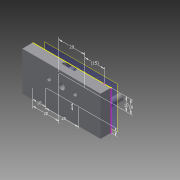
# Autodesk Inventor part: detalKKoretke
Saved by Autodesk Inventor 2015 (Build 190159000, 159)
## iProperties
Created: 2016-04-08
Part Number: detalKKoretke
Material: Generic
Document SubType Name: Modeling
Designer: Andreas
Density: 1 g/cm^3
Appearance: Default
Author: Andreas
Autodesk Inventor part; units mm, degrees
ref_plane "YZ Plane" through (0, 0, 0) normal (1, 0, 0) x (0, 1, 0)
ref_plane "XZ Plane" through (0, 0, 0) normal (0, 1, 0) x (-1, 0, 0)
ref_plane "XY Plane" through (0, 0, 0) normal (0, 0, 1) x (1, 0, 0)
sketch "Sketch1" plane through (0, 0, 0) normal (0, 1, 0) x (-1, 0, 0)
  line L0 (0, 0) -> (60, 0)
  line L1 (60, 0) -> (60, -30)
  line L2 (60, -30) -> (0, -30)
  line L3 (0, -30) -> (0, 0)
  dimension "d0" = 60
  dimension "d1" = 30
  dimension "d2" = 60
  constraints: 8 end point, 2 perpendicular, 1 horizontal
  measures "d0" distance of L0.start L0.end
  measures "d1" distance of L0.end L1.end
  measures "d2" distance of L1.end L2.end
extrude "Extrusion1" add sketch "Sketch1" against normal blind 5 and the other way blind 3
sketch "Sketch2" plane through (0, 3, 0) normal (0, 1, 0) x (1, 0, 0)
  line L0 (-60, 30) -> (-60, 0) projected
  line L1 (0, 0) -> (0, 30) projected
  line L2 (0, 30) -> (-60, 30) projected
  line L3 (-60, 0) -> (0, 0) projected
  line L4 (-5, 0) -> (-5, 30) projected
  point P0 (-40, 10)
  point P1 (-20, 10)
  dimension "d44" = 10
  dimension "d45" = 20
  dimension "d46" = 20
  dimension "d47" = 10
  dimension "d67" = 15
  measures "d44" distance from line of L3 point (-40, 10)
  measures "d45" distance from line of L0 point (-40, 10)
  measures "d46" distance of point (-40, 10) point (-20, 10)
  measures "d47" distance from line of L3 point (-20, 10)
  measures "d67" distance from line of L4 point (-20, 10)
sketch "Sketch3" plane through (0, 3, 0) normal (0, 1, 0) x (1, 0, 0)
  line L0 (0, 30) -> (-60, 30) projected
  line L1 (-60, 0) -> (-60, 30) projected
  point P0 (0, 0)
  point P1 (-50, 25)
  point P2 (-5, 30)
  point P3 (-25, 25)
  dimension "d56" = 5
  dimension "d57" = 10
  dimension "d58" = 25
  dimension "d59" = 5
  measures "d56" distance from line of L0 point (-50, 25)
  measures "d57" distance from line of L1 point (-50, 25)
  measures "d58" distance of point (-50, 25) point (-25, 25)
  measures "d59" distance from line of L0 point (-25, 25)
sketch "Sketch11" plane through (0, 3, 0) normal (0, 1, 0) x (1, 0, 0)
  point P0 (-20, 10)
  point P1 (-40, 10)
hole "Hole2" at (-20, 3, -10) at (-40, 3, -10) direction (0, -1, 0) diameter 3.4 depth 8
sketch "Sketch16" plane through (-60, -5, 0) normal (0, 0, 1) x (1, 0, 0)
  line L0 (60, 8) -> (0, 8) projected
  line L1 (25, 8) -> (26, 8)
  line L2 (26, 8) -> (26, 7)
  line L3 (26, 7) -> (25, 7)
  line L4 (25, 7) -> (25, 5)
  line L5 (25, 5) -> (35, 5)
  line L6 (35, 5) -> (35, 7)
  line L7 (35, 7) -> (34, 7)
  line L8 (34, 7) -> (34, 8)
  line L9 (35, 8) -> (25, 8)
  point P0 (60, 5)
  dimension "d90" = 1
  dimension "d91" = 1
  dimension "d92" = 2
  dimension "d93" = 10
  dimension "d94" = 1
  constraints: 18 end point, 7 point on line, 6 perpendicular, 1 collinear
  measures "d90" distance of L1.start L1.end
  measures "d91" distance of L1.end L2.end
  measures "d92" distance of L3.end L4.end
  measures "d93" distance of L4.end L5.end
  measures "d94" distance of L6.end L7.end
extrude "Extrusion6" cut sketch "Sketch16" against normal up to next
sketch "Sketch17" plane through (-35, 0, 0) normal (0, 1, 0) x (1, 0, 0)
  circle A0 centre (5, 10) radius 2.5
  point P0 (35, 0)
  dimension "d97" = 5
  constraints: 1 centre point
  measures "d97" diameter of A0
extrude "Extrusion7" cut sketch "Sketch17" against normal up to next
sketch "Sketch18" plane through (0, 3, 0) normal (0, 1, 0) x (1, 0, 0)
  circle A0 centre (-12, 22) radius 2.5
  circle A1 centre (-48, 22) radius 2.5
  line L0 (-60, 30) -> (-60, 0) projected
  line L1 (0, 0) -> (0, 30) projected
  line L2 (-26, 0) -> (0, 0) projected
  line L3 (-60, 0) -> (-34, 0) projected
  dimension "d100" = 5
  dimension "d101" = 5
  dimension "d107" = 12
  dimension "d108" = 12
  dimension "d122" = 22
  dimension "d123" = 22
  constraints: 2 centre point
  measures "d100" diameter of A0
  measures "d101" diameter of A1
  measures "d107" distance from line of L0 A1.centre
  measures "d108" distance from line of L1 A0.centre
  measures "d122" distance from line of L2 A0.centre
  measures "d123" distance from line of L3 A1.centre
extrude "Extrusion8" add sketch "Sketch18" along normal blind 19
ref_plane "Work Plane2" through (0, 6.5, 0) normal (0, 1, 0) x (1, 0, 0)
sketch "Sketch19" plane through (0, 6.5, 0) normal (0, 1, 0) x (1, 0, 0)
  circle A0 centre (-48, 22) radius 2.5 projected
  circle A1 centre (-48, 22) radius 3.5
  circle A2 centre (-12, 22) radius 3.5
  line L0 (0, 0) -> (0, 30) projected
  line L1 (-26, 0) -> (0, 0) projected
  dimension "d105" = 7
  dimension "d106" = 7
  dimension "d109" = 12
  dimension "d124" = 22
  constraints: 2 centre point, 1 coincident
  measures "d105" diameter of A1
  measures "d106" diameter of A2
  measures "d109" distance from line of L0 A2.centre
  measures "d124" distance from line of L1 A2.centre
extrude "Extrusion9" add sketch "Sketch19" along normal blind 1.25 and the other way blind 3.5
sketch "Sketch20" plane through (-12, 22, -22) normal (0, 1, 0) x (1, 0, 0)
  circle A0 centre (0, 0) radius 1
  circle A1 centre (-36, 0) radius 2.5 projected
  circle A2 centre (-36, 0) radius 1
  point P0 (12, -22)
  dimension "d114" = 2
  dimension "d115" = 2
  constraints: 2 centre point, 1 coincident
  measures "d114" diameter of A0
  measures "d115" diameter of A2
extrude "Extrusion10" cut sketch "Sketch20" against normal blind 4 contours A0 | A2
thread "Thread1" size "M2x0.4" class "6H" standard "ANSI Metric M Profile" full length
thread "Thread2" size "M2x0.4" class "6H" standard "ANSI Metric M Profile" full length
body "Solid1"
